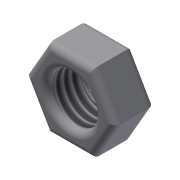
# Autodesk Inventor part: m6nut
Saved by Autodesk Inventor 2015 (Build 190159000, 159)
## iProperties
Created: 2015-10-28
Part Number: m6nut
Material: Generic
Document SubType Name: Modeling
Designer: jad211
Density: 1 g/cm^3
Appearance: Default
Author: jad211
Autodesk Inventor part; units mm, degrees
ref_plane "YZ Plane" through (0, 0, 0) normal (1, 0, 0) x (0, 1, 0)
sketch "Sketch1" plane through (0, 0, 0) normal (0, 1, 0) x (-1, 0, 0)
  line L0 (2.8251, -4.9022) -> (-2.8329, -4.8978)
  line L1 (-2.8329, -4.8978) -> (-5.658, 0.0045)
  line L2 (-5.658, 0.0045) -> (-2.8251, 4.9022)
  line L3 (-2.8251, 4.9022) -> (2.8329, 4.8978)
  line L4 (2.8329, 4.8978) -> (5.658, -0.0045)
  line L5 (5.658, -0.0045) -> (2.8251, -4.9022)
  circle A0 centre (0, 0) radius 3
  dimension "d0" = 9.8
  dimension "d1" = 6
  constraints: 12 end point, 2 coincident, 1 centre point, 13 other
  measures "d0" distance between parallel lines of L0 L3
  measures "d1" diameter of A0
extrude "Extrusion1" add sketch "Sketch1" along normal blind 5
fillet "Fillet1" radius 0.8 14 edges at (4.2416, 5, 2.4533) (4.2455, 5, -2.4467) (0.0039, 5, -4.9) (-4.2416, 5, -2.4533) (-4.2455, 5, 2.4467) (-0.0039, 5, 4.9) (-0.0039, 0, 4.9) (4.2416, 0, 2.4533) (4.2455, 0, -2.4467) (0.0039, 0, -4.9) (-4.2416, 0, -2.4533) (-4.2455, 0, 2.4467) (3, 5, 0) (3, 0, 0)
thread "Thread1" size "M6x1" class "6H" standard "ANSI Metric M Profile" full length
ref_plane "Work Plane1" through (0, 5, 0) normal (0, 1, 0) x (1, 0, 0)
ref_plane "Work Plane2" through (0, 0, 0) normal (0, -1, 0) x (1, 0, 0)
body "Solid1"
